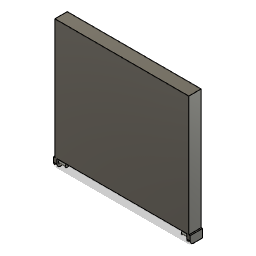
door (Autodesk Fusion 360 design; units mm, degrees)
Autodesk Fusion 360 part; units mm, degrees
note: some values were not read from the file. Set by a fixed rule: which sketch regions a step uses.
sketch "Sketch1" plane through (0, 0, 0) normal (0, 0, 1) x (1, 0, 0)
  line L0 (-14, 0) -> (175, 0)
  line L1 (180, -12) -> (180, 0)
  line L2 (178, 175) -> (-17, 175)
  line L3 (-19, 0) -> (-19, -12)
  line L4 (-19, -12) -> (-14, -12)
  line L5 (-14, -12) -> (-14, 0)
  line L6 (180, -12) -> (175, -12)
  line L7 (175, -12) -> (175, 0)
  line L8 (180, 0) -> (178, 0)
  line L9 (178, 0) -> (178, 175)
  line L10 (-17, 0) -> (-17, 175)
  line L11 (-17, 0) -> (-19, 0)
  dimension "d1" = 189
  dimension "d13" = 12
  dimension "d14" = 12
  dimension "d16" = 5
  dimension "d24" = 175
  dimension "d31" = 2
  dimension "d32" = 5
  dimension "d33" = 2
  constraint horizontal L0
  constraint vertical L1
  constraint perpendicular L2 L3
  constraint perpendicular L3 L4
  constraint perpendicular L0 L5
  constraint perpendicular L1 L6
  constraint perpendicular L0 L7
  constraint coincident L1.end L8.start
  constraint perpendicular L1 L8
  constraint perpendicular L2 L9
  constraint perpendicular L2 L10
  constraint perpendicular L3 L11
  measures "d1" distance of L0.start L0.end
  measures "d13" distance of L0.end L6.end
  measures "d14" distance of L0.start L4.end
  measures "d16" distance of L1.start L6.end
  measures "d24" distance of L0 L2
  measures "d31" distance of L1.end L8.end
  measures "d32" distance of L3.end L4.end
  measures "d33" distance of L10.start L3.start
extrude "Extrude1" add sketch "Sketch1" along normal blind 10
sketch "Sketch2" plane through (-14, 0, 0) normal (1, 0, 0) x (0, 0, -1)
  line L0 (0, -12) -> (0, 0)
  line L1 (0, 0) -> (-10, 0)
  line L2 (-10, 0) -> (-10, -12)
  line L3 (-10, -12) -> (0, -12)
  circle A0 centre (-5, -5.6) radius 2.9
  dimension "d5" = 5.8
  dimension "d6" = 5.6
  measures "d5" diameter of A0
  measures "d6" distance of L1 A0.centre
extrude "Extrude2" add sketch "Sketch2" along normal blind 10 contours A0
sketch "Sketch3" plane through (175, 0, 0) normal (-1, 0, 0) x (0, 0, 1)
  line L0 (0, 0) -> (0, -12)
  line L1 (0, -12) -> (10, -12)
  line L2 (10, -12) -> (10, 0)
  line L3 (10, 0) -> (0, 0)
  circle A0 centre (5, -5.6) radius 2.9
  dimension "d9" = 5.8
  dimension "d10" = 5.6
  measures "d9" diameter of A0
  measures "d10" distance of L3 A0.centre
extrude "Extrude3" add sketch "Sketch3" along normal blind 10 contours A0
sketch "Sketch4" plane through (0, 0, 0) normal (0, 0, -1) x (-1, 0, 0)
  line L0 (19, -12) -> (19, 0)
  line L1 (17, 0) -> (17, 175)
  line L2 (17, 175) -> (-178, 175)
  line L3 (-178, 175) -> (-178, 0)
  line L4 (-178, 0) -> (-180, 0)
  line L5 (-180, 0) -> (-180, -12)
  line L6 (-180, -12) -> (-175, -12)
  line L7 (-175, -12) -> (-175, 0)
  line L8 (-175, 0) -> (14, 0)
  line L9 (14, 0) -> (14, -12)
  line L10 (14, -12) -> (19, -12)
  line L11 (-178, 0) -> (-180, 0)
  line L12 (-180, 0) -> (-180, -12)
  line L13 (-180, -12) -> (-175, -12)
  line L14 (-175, -12) -> (-175, 172)
  line L15 (-175, 172) -> (14, 172)
  line L16 (14, 172) -> (14, -12)
  line L17 (14, -12) -> (19, -12)
  line L18 (19, -12) -> (19, 0)
  line L19 (19, 0) -> (17, 0)
  line L20 (17, 0) -> (17, 175)
  line L21 (17, 175) -> (-178, 175)
  line L22 (-178, 175) -> (-178, 0)
  line L23 (19, 0) -> (17, 0)
  dimension "d19" = 3
  dimension "d20" = 3
  dimension "d21" = 3
  constraint coincident L3.end L4.start
  constraint coincident L4.end L5.start
  constraint coincident L5.end L6.start
  constraint coincident L6 L7.start
  constraint perpendicular L6 L14
  constraint perpendicular L3 L15
  constraint perpendicular L8 L16
  constraint coincident L10 L9.end
  constraint coincident L0.start L10.end
  constraint coincident L0.end L18.end
  constraint coincident L1.start L19.end
  constraint coincident L1.end L2.start
  constraint coincident L2.end L3.start
  measures "d19" distance of L16 L20
  measures "d20" distance of L14 L22
  measures "d21" distance of L15 L21
extrude "Extrude4" add sketch "Sketch4" along normal blind 8 contours L0 L1 L2 L3 L4 L5 L6 L7 L9 L10 L11 L12 L13 L14 L15 L16 L17 L18 L19 L20 L21 L22 L23
fillet "Fillet1" radius 5 1 edges at (-16.5, -12, 10)
fillet "Fillet2" radius 5 1 edges at (177.5, -12, 10)
extrude "Extrude5" cut 1 faces at (112, 114.6667, 0) along direction (0, 0, 1) blind 2
